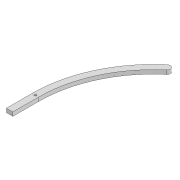
# Autodesk Inventor part: Part_11
Saved by Autodesk Inventor 2022 (Build 260153000, 153)
## iProperties
Created: 2022-04-23
Part Number: Part_11
Material: Generic
Document SubType Name: Modeling
Designer: dell
Density: 1 g/cm^3
Appearance: Default
Author: dell
Autodesk Inventor part; units mm, degrees
ref_plane "YZ Plane" through (0, 0, 0) normal (1, 0, 0) x (0, 1, 0)
ref_plane "XZ Plane" through (0, 0, 0) normal (0, 1, 0) x (-1, 0, 0)
ref_plane "XY Plane" through (0, 0, 0) normal (0, 0, 1) x (1, 0, 0)
sketch "Sketch1" plane through (0, 0, 0) normal (0, 1, 0) x (-1, 0, 0)
  line L0 (0, 0) -> (10, 0)
  line L1 (10, 0) -> (10, -40)
  line L2 (10, -40) -> (0, -40)
  line L3 (0, -40) -> (0, 0)
  circle A0 centre (5, -40) radius 5
  arc A1 (-63.2267, -176.1805) -> (0, -40) centre (-178.2692, -40) ccw
  arc A2 (-56.7733, -183.8195) -> (10, -40) centre (-178.2692, -40) ccw
  circle A3 centre (-60, -180) radius 5
  circle A4 centre (5, -40) radius 1.65
  dimension "d1" = 10
  dimension "d0" = 10
  dimension "d3" = 40
  dimension "d4" = 10
  dimension "d6" = 180
  dimension "d7" = 60
  dimension "d8" = 3.3
  constraints: 8 end point, 6 point on circle, 4 centre point, 2 parallel, 2 tangent, 1 coincident, 1 horizontal, 1 horizontal alignment, 1 midpoint, 1 perpendicular, 1 point on line, 4 other
  measures "d0" distance between parallel lines of L3 L1
  measures "d3" distance between parallel lines of L0 L2
  measures "d4" diameter of A3
  measures "d6" distance from line of L0 A3.centre
  measures "d7" horizontal distance of L0.start A3.centre
  measures "d8" diameter of A4
extrude "Extrusion1" add sketch "Sketch1" along normal blind 6 contours L0 L1 A0 L3 | A0 L2 A4 | L2 A4 A0 | A0 A2 A3 A1 | A3
body "Solid1"
